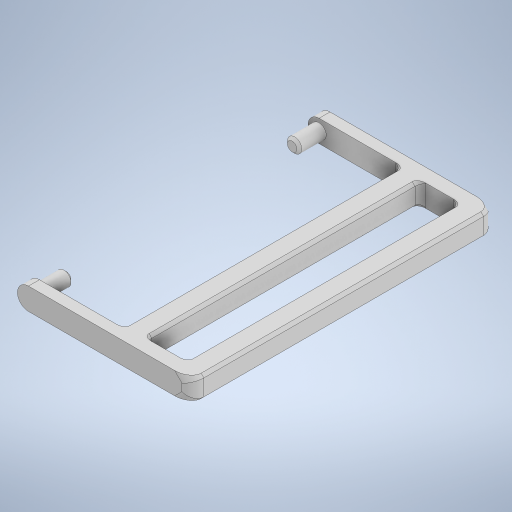
# Autodesk Inventor part: LI0007-LATCH
Saved by Autodesk Inventor 2023 (Build 270158000, 158)
## iProperties
Created: 2023-03-15
Part Number: LI0007-LATCH
Material: Generic
Document SubType Name: Modeling
Designer: Louis
Density: 1 g/cm^3
Appearance: Default
Author: Louis
Autodesk Inventor part; units mm, degrees
ref_plane "YZ Plane" through (0, 0, 0) normal (1, 0, 0) x (0, 1, 0)
ref_plane "XZ Plane" through (0, 0, 0) normal (0, 1, 0) x (-1, 0, 0)
ref_plane "XY Plane" through (0, 0, 0) normal (0, 0, 1) x (1, 0, 0)
sketch "Sketch1" plane through (0, 0, 0) normal (0, 0, 1) x (1, 0, 0)
  line L0 (-16, 4) -> (16, 4)
  line L1 (16, 4) -> (16, 0)
  line L2 (16, 0) -> (-16, 0)
  line L3 (-16, 0) -> (-16, 4)
  point P0 (0, 0)
  point P1 (0, 0)
  dimension "d0" = 4
  dimension "d1" = 32
  constraints: 8 end point, 2 coincident, 2 parallel, 1 horizontal, 1 midpoint, 1 perpendicular
  measures "d0" distance of L0.end L1.end
  measures "d1" distance of L0.start L0.end
extrude "Extrusion1" add sketch "Sketch1" along normal mid plane 55
sketch "Sketch2" plane through (0, 0, 0) normal (0, 0, 1) x (1, 0, 0)
  line L0 (-16, 4) -> (-16, 0) projected
  line L1 (-16, 4) -> (1, 4)
  line L2 (0, 0) -> (-16, 0)
  line L3 (-16, 0) -> (-16, 4)
  line L4 (1, 4) -> (1, 0)
  line L5 (0, 0) -> (1, 0)
  dimension "d22" = 1
  constraints: 10 end point, 2 horizontal, 2 parallel, 1 vertical
  measures "d22" distance from line of L2.start L4
extrude "Extrusion2" cut sketch "Sketch2" along normal mid plane 51
sketch "Sketch3" plane through (0, 0, -25.5) normal (0, 0, 1) x (1, 0, 0)
  circle A0 centre (-14, 2) radius 1.4
  line L0 (-16, 0) -> (-16, 4) projected
  point P0 (0, 0)
  point P1 (-16, 2)
  dimension "d6" = 2.8
  dimension "d7" = 2
  constraints: 1 centre point, 1 horizontal alignment, 1 midpoint
  measures "d6" diameter of A0
  measures "d7" distance from line of L0 A0.centre
extrude "Extrusion3" add sketch "Sketch3" along normal blind 5
mirror "Mirror1" about plane through (0, 0, 0) normal (0, 0, 1) of "Extrusion3"
sketch "Sketch4" plane through (0, 0, 0) normal (0, 0, 1) x (1, 0, 0)
  line L0 (16, 4) -> (-16, 4) projected
  line L1 (-16, 0) -> (16, 0) projected
  line L2 (12, 4) -> (5, 4)
  line L3 (5, 4) -> (5, 0)
  line L4 (5, 0) -> (12, 0)
  line L5 (12, 0) -> (12, 4)
  point P0 (0, 0)
  point P1 (0, 4)
  point P2 (12, 0)
  point P3 (0, 0)
  dimension "d10" = 4
  dimension "d23" = 5
  constraints: 8 end point, 2 parallel, 2 point on line, 1 horizontal, 1 midpoint, 1 perpendicular
  measures "d10" distance of L0.start L2.start
  measures "d23" distance from line of point (0, 0) L3
extrude "Extrusion4" cut sketch "Sketch4" along normal mid plane 50
chamfer "Chamfer1" distance 0.5 angle 45 10 edges at (12, 4, 0) (12, 0, 0) (16, 4, 0) (16, 0, 0) (5, 4, 0) (5, 0, 0) (-15.4, 2, -20.5) (-15.4, 2, 20.5) (1, 4, 0) (1, 0, 0)
fillet "Fillet1" radius 2 10 edges at (-16, 4, -26.5) (-16, 0, -26.5) (-16, 4, 26.5) (-16, 0, 26.5) (15.75, 3.75, 27.5) (15.75, 0.25, 27.5) (16, 2, -27.5) (16, 2, 27.5) (15.75, 3.75, -27.5) (15.75, 0.25, -27.5)
fillet "Fillet3" radius 1 18 edges at (12, 2, -25) (12.25, 3.75, -25) (12.25, 0.25, -25) (4.75, 0.25, -25) (5, 2, -25) (4.75, 3.75, -25) (5, 2, 25) (4.75, 3.75, 25) (4.75, 0.25, 25) (12.25, 0.25, 25) (12, 2, 25) (12.25, 3.75, 25) (1.25, 3.75, -25.5) (1, 2, -25.5) (1.25, 0.25, -25.5) (1.25, 0.25, 25.5) (1, 2, 25.5) (1.25, 3.75, 25.5)
thicken "Thicken1" operation cut thickness 0.1 both sides no extend neighbours no toward (-0.9967573, 0.0804666, 0) faces at (-12.6045, 1.8873, -22.5) (-12.8025, 1.7048, -20.8333) (-13.7087, 2.3261, -20.5)
thicken "Thicken2" operation cut thickness 0.1 both sides no extend neighbours no toward (-0.9967573, 0.0804666, 0) faces at (-12.6045, 1.8873, 22.5) (-12.8025, 1.7048, 20.8333) (-13.7087, 2.3261, 20.5)
body "Solid1"
